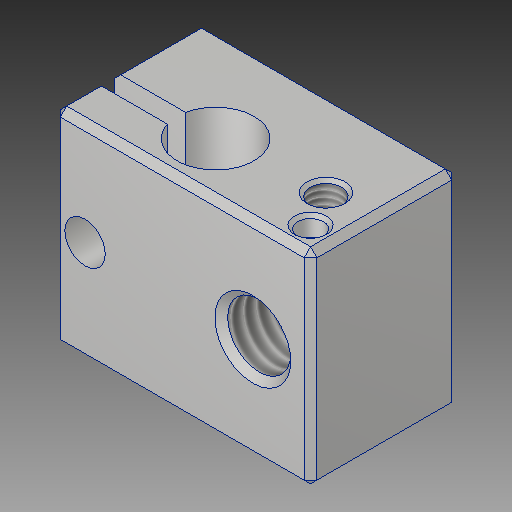
# Autodesk Inventor part: Bloque de chauffe
Saved by Autodesk Inventor 2017 (Build 210142000, 142)
## iProperties
Company: FABLAB Frenchmakers
Part Number: Bloque de chauffe
Material: Aluminium
Document SubType Name: Modeling
Designer: FABLAB Frenchmakers
Density: 2.7 g/cm^3
Appearance: Aluminium - Plat(2)
Mass: 7.45253 g
Surface Area: 20.1662 cm^2
Volume: 2.7602 cm^3
Project: 1420 Vauban 3D XL
Catalog Web Link: http://frenchmakers.com/
Stock Number: 1420-02-22
Autodesk Inventor part; units mm, degrees
ref_plane "YZ Plane" through (0, 0, 0) normal (1, 0, 0) x (0, 1, 0)
ref_plane "XZ Plane" through (0, 0, 0) normal (0, 1, 0) x (-1, 0, 0)
ref_plane "XY Plane" through (0, 0, 0) normal (0, 0, 1) x (1, 0, 0)
sketch "Esquisse1" plane through (0, 0, 0) normal (0, 0, 1) x (1, 0, 0)
  line L0 (-10, -8) -> (10, -8)
  line L1 (10, -8) -> (10, 8)
  line L2 (10, 8) -> (-10, 8)
  line L3 (-10, 8) -> (-10, -8)
  line L4 (-10, -8) -> (10, 8) construction
  line L5 (10, -8) -> (-10, 8) construction
  point P0 (0, 0)
  dimension "d0" = 20
  dimension "d1" = 16
  constraints: 12 end point, 2 midpoint, 2 parallel, 1 horizontal, 1 perpendicular
  measures "d0" distance of L1.end L2.end
  measures "d1" distance of L0.end L1.end
extrude "Extrusion1" add sketch "Esquisse1" along normal mid plane 11.5
sketch "Esquisse2" plane through (0, 0, 5.75) normal (0, 0, 1) x (1, 0, 0)
  line L0 (10, -8) -> (10, 8) projected
  point P0 (0, 0)
  point P1 (5.5, 0)
  dimension "d14" = 5.5
  constraints: 1 horizontal alignment
  measures "d14" distance of point (0, 0) point (5.5, 0)
hole "Perçage1" at (5.5, 0, 5.75) direction (0, 0, -1) diameter 4.917 depth 17.1 tip angle 118 thread size "M6x1" class "6H" standard "ISO Metric profile"
chamfer "Chanfrein1" distance 0.5 angle 45 2 edges at (5.5, 2.4585, 5.75) (5.5, 2.4585, -5.75)
chamfer "Chanfrein2" distance 0.5 angle 45 12 edges at (-10, 8, 0) (-10, 0, 5.75) (0, 8, 5.75) (-10, -8, 0) (-10, 0, -5.75) (0, -8, -5.75) (0, -8, 5.75) (10, -8, 0) (10, 0, 5.75) (10, 0, -5.75) (10, 8, 0) (0, 8, -5.75)
sketch "Esquisse3" plane through (-10, -8, 5.75) normal (0, -1, 0) x (1, 0, 0)
  arc A0 (5.5606, -4.7) -> (5.6382, -3.2) centre (8.5, -4.1) ccw
  line L0 (0, -4.7) -> (5.5606, -4.7)
  line L1 (5.6382, -3.2) -> (0, -3.2)
  line L2 (0, -3.2) -> (0, -4.7)
  line L3 (20, -11.5) -> (20, 0) construction
  line L4 (0, 0) -> (20, 0) construction
  line L5 (0, 0) -> (0, -11.5) construction
  point P0 (10, -5.75)
  dimension "d18" = 6
  dimension "d19" = 11.5
  dimension "d20" = 4.1
  dimension "d21" = 1.5
  dimension "d22" = 3.2
  constraints: 6 end point, 2 point on circle, 1 centre point, 1 collinear, 1 horizontal, 1 parallel
  measures "d18" diameter of A0
  measures "d19" distance from line of L3 A0.centre
  measures "d20" distance from line of L4 A0.centre
  measures "d21" distance between parallel lines of L1 L0
  measures "d22" distance between parallel lines of L4 L1
extrude "Extrusion2" cut sketch "Esquisse3" against normal through all
sketch "Esquisse4" plane through (0, 0, 5.75) normal (0, 0, 1) x (1, 0, 0)
  line L0 (-10, 8) -> (-10, -8) projected
  point P0 (0, 0)
  point P1 (-7.575, 0)
  dimension "d25" = 2.425
  constraints: 1 horizontal alignment
  measures "d25" distance from line of L0 point (-7.575, 0)
hole "Perçage2" at (-7.575, 0, 5.75) direction (0, 0, -1) diameter 2.459 end through all counterbore diameter 3.15 counterbore depth 4 thread size "M3x0.5" class "6H" standard "ISO Metric profile"
sketch "Esquisse5" plane through (-9.5, 8, 5.25) normal (0, 1, 0) x (1, 0, 0)
  line L0 (19.5, 0) -> (19.5, 10.5) projected
  line L1 (0, -0.5) -> (19, -0.5) projected
  point P0 (9.5, 5.25)
  point P1 (15.95, 4.25)
  dimension "d36" = 3.55
  dimension "d37" = 4.75
  measures "d36" distance from line of L0 point (15.95, 4.25)
  measures "d37" distance from line of L1 point (15.95, 4.25)
hole "Perçage3" at (6.45, 8, 1) direction (0, -1, 0) diameter 2.459 depth 5 tip angle 118 thread size "M3x0.5" class "6H" standard "ISO Metric profile"
sketch "Esquisse6" plane through (-9.5, 8, 5.25) normal (0, 1, 0) x (1, 0, 0)
  line L0 (0, -0.5) -> (19, -0.5) projected
  line L1 (19.5, 0) -> (19.5, 10.5) projected
  point P0 (9.5, 5.25)
  point P1 (17.55, 1.45)
  dimension "d45" = 1.95
  dimension "d46" = 1.95
  measures "d45" distance from line of L0 point (17.55, 1.45)
  measures "d46" distance from line of L1 point (17.55, 1.45)
hole "Perçage4" at (8.05, 8, 3.8) direction (0, -1, 0) diameter 1 depth 4 tip angle 118 counterbore diameter 2 counterbore depth 1.5
chamfer "Chanfrein3" distance 0.25 angle 45 2 edges at (8.05, 8, 2.8) (6.45, 8, -0.2295)
equation "\"d46\" = d45"
